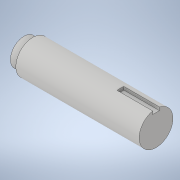
# Autodesk Inventor part: MotorShaft
Saved by Autodesk Inventor 2021 (Build 250183000, 183)
## iProperties
Created: 2020-09-20
Part Number: MotorShaft
Material: Generic
Document SubType Name: Modeling
Designer: PhotonUser
Density: 1 g/cm^3
Appearance: Default
Author: PhotonUser
Autodesk Inventor part; units mm, degrees
ref_plane "YZ Plane" through (0, 0, 0) normal (1, 0, 0) x (0, 1, 0)
ref_plane "XZ Plane" through (0, 0, 0) normal (0, 1, 0) x (-1, 0, 0)
ref_plane "XY Plane" through (0, 0, 0) normal (0, 0, 1) x (1, 0, 0)
sketch "Sketch1" plane through (0, 0, 0) normal (1, 0, 0) x (0, 1, 0)
  circle A0 centre (0, 0) radius 15.875
  dimension "d0" = 31.75
  constraints: 1 centre point, 1 coincident
  measures "d0" diameter of A0
extrude "Extrusion1" add sketch "Sketch1" along normal blind 123.952
ref_plane "Work Plane1" through (71.7931, 0, 0) normal (1, 0, 0) x (0, 0, -1)
sketch "Sketch9" plane through (123.952, 0, 0) normal (1, 0, 0) x (0, 0, -1)
  line L0 (-3.175, 15.875) -> (-3.175, 12.7)
  line L1 (-3.175, 12.7) -> (3.175, 12.7)
  line L2 (3.175, 12.7) -> (3.175, 15.875)
  line L3 (0, 0) -> (0, 19.977)
  circle A0 centre (0, 0) radius 15.875 projected
  line L4 (0, 15.875) -> (-16.159, 15.875)
  point P0 (0, 12.7)
  point P1 (3.175, 15.5543)
  point P2 (-3.175, 15.5543)
  dimension "d26" = 6.35
  dimension "d27" = 3.175
  constraints: 10 end point, 2 horizontal, 2 perpendicular, 2 point on line, 2 vertical, 1 midpoint, 1 parallel, 2 other
  measures "d26" distance of L0.end L1.end
  measures "d27" distance between parallel lines of L1 L4
extrude "Extrusion9" cut sketch "Sketch9" against normal blind 33.3502 contours A0 L3 L1 L0 | A0 L2 L1 L3
sketch "Sketch10" plane through (0, 0, 0) normal (-1, 0, 0) x (0, 0, 1)
  circle A0 centre (0, 0) radius 15.875
  circle A1 centre (0, 0) radius 12.7
  dimension "d30" = 25.4
  constraints: 2 centre point, 2 coincident
  measures "d30" diameter of A1
extrude "Extrusion10" cut sketch "Sketch10" against normal blind 8.255
body "Solid1"
